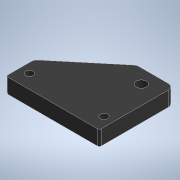
# Autodesk Inventor part: 21_X_Pulley_holder
Saved by Autodesk Inventor 2022.2 (Build 262287010, 287A)
## iProperties
Created: 2022-04-30
Part Number: 21_X_Pulley_holder
Material: PET-Kunststoff
Document SubType Name: Modeling
Designer: MXBD
Density: 1.541 g/cm^3
Appearance: Gummi - Schwarz
Author: MXBD
Autodesk Inventor part; units mm, degrees
ref_plane "YZ Plane" through (0, 0, 0) normal (1, 0, 0) x (0, 1, 0)
ref_plane "XZ Plane" through (0, 0, 0) normal (0, 1, 0) x (-1, 0, 0)
ref_plane "XY Plane" through (0, 0, 0) normal (0, 0, 1) x (1, 0, 0)
sketch "Skizze1" plane through (0, 0, 0) normal (0, 1, 0) x (-1, 0, 0)
  line L0 (0, -48) -> (0, 8) projected
  line L1 (-10, 0) -> (60, 0) projected
  line L2 (12.9651, 0) -> (0, 0)
  line L3 (0, 0) -> (0, -40)
  line L4 (0, -40) -> (20, -40)
  line L5 (20, -40) -> (20, -15)
  line L6 (20, -15) -> (50, -15)
  line L7 (50, -15) -> (50, 0)
  line L8 (50, 0) -> (12.9651, 0)
  dimension "d0" = 40
  dimension "d1" = 15
  dimension "d2" = 50
  dimension "d5" = 20
  constraints: 14 end point, 3 perpendicular, 3 point on line, 2 collinear, 1 horizontal
  measures "d0" distance between parallel lines of L1 L4
  measures "d1" distance between parallel lines of L1 L6
  measures "d2" distance between parallel lines of L0 L7
  measures "d5" distance between parallel lines of L5 L3
extrude "Extrusion1" add sketch "Skizze1" along normal blind 8
sketch "Skizze2" plane through (0, 8, 0) normal (0, 1, 0) x (1, 0, 0)
  line L0 (-50, 15) -> (-50, 0) construction
  line L1 (-50, 7.5) -> (0, 7.5) construction
  line L2 (0, 0) -> (0, 40) construction
  point P0 (-45, 7.5)
  point P1 (-5, 7.5)
  dimension "d8" = 40
  dimension "d9" = 5
  constraints: 3 point on line, 2 end point, 1 horizontal, 1 midpoint
  measures "d8" distance of point (-5, 7.5) point (-45, 7.5)
  measures "d9" distance from line of L2 point (-5, 7.5)
hole "Bohrung1" at (-45, 8, -7.5) at (-5, 8, -7.5) direction (0, -1, 0) diameter 4 end through all
sketch "Skizze3" plane through (0, 8, 0) normal (0, 1, 0) x (1, 0, 0)
  line L0 (0, 40) -> (-20, 40) construction
  line L1 (-10, 40) -> (-10, 0) construction
  line L2 (-50, 0) -> (0, 0) construction
  line L3 (-20, 40) -> (-20, 15) construction
  point P0 (-10, 32.5)
  dimension "d24" = 7.5
  constraints: 2 end point, 1 midpoint, 1 point on line, 1 vertical
  measures "d24" distance from line of L0 point (-10, 32.5)
hole "Bohrung2" at (-10, 8, -32.5) direction (0, -1, 0) diameter 5.5 end through all clearance for "Inbusschraube ISO 4762" size "M5" standard "ISO"
sketch "Skizze4" plane through (0, 8, 0) normal (0, 1, 0) x (1, 0, 0)
  line L0 (0, 40) -> (-20, 40) projected
  line L1 (-50, 15) -> (-50, 0) projected
  line L2 (-20, 40) -> (-50, 15)
  line L3 (-50, 15) -> (-20, 15)
  line L4 (-20, 40) -> (-20, 15) projected
  line L5 (-20, 15) -> (-20, 40)
  point P0 (0, 0)
  constraints: 6 end point, 1 collinear, 1 perpendicular
extrude "Extrusion2" add sketch "Skizze4" against normal up to surface (8 mm away)
fillet "Rundung2" radius 1 2 edges at (0, 4, 0) (-50, 4, 0)
fillet "Rundung3" radius 3 3 edges at (0, 4, -40) (-20, 4, -40) (-50, 4, -15)
